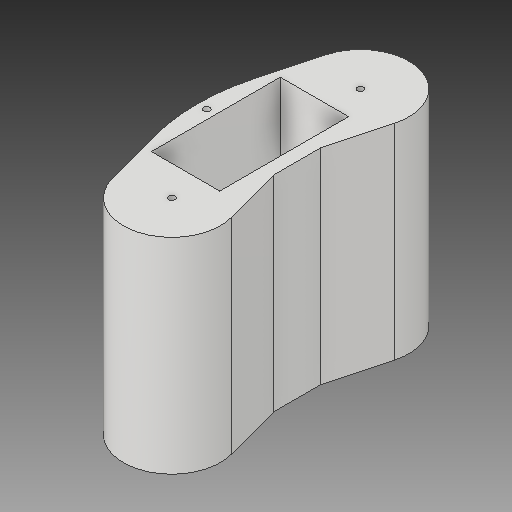
# Autodesk Inventor part: TA001
Saved by Autodesk Inventor 2017 SP1 (Build 210196100, 196)
## iProperties
Created: 2017-09-22
Part Number: TA001
Material: ABS Plastic
Document SubType Name: Modeling
Designer: Zach
Density: 1.06 g/cm^3
Appearance: CR White
Mass: 16966 g
Surface Area: 7360.25 cm^2
Volume: 16005.6 cm^3
Author: Zach
Autodesk Inventor part; units mm, degrees
ref_plane "YZ Plane" through (0, 0, 0) normal (1, 0, 0) x (0, 1, 0)
ref_plane "XZ Plane" through (0, 0, 0) normal (0, 1, 0) x (-1, 0, 0)
ref_plane "XY Plane" through (0, 0, 0) normal (0, 0, 1) x (1, 0, 0)
sketch "Sketch2" plane through (0, 0, 0) normal (0, 1, 0) x (-1, 0, 0)
  circle A0 centre (0, 0) radius 80 construction
  line L0 (77.2741, 20.7055) -> (103.156, -75.8871)
  line L1 (-77.2741, -20.7055) -> (-51.3922, -117.2981)
  line L2 (103.156, -75.8871) -> (-51.3922, -117.2981) construction
  line L3 (103.156, -75.8871) -> (103.156, -235.8871) construction
  line L4 (103.156, -235.8871) -> (-51.3922, -194.476) construction
  line L5 (-51.3922, -117.2981) -> (-51.3922, -194.476)
  circle A1 centre (0, -311.7741) radius 80 construction
  line L6 (-51.3922, -194.476) -> (-77.2741, -291.0686)
  line L7 (103.156, -235.8871) -> (77.2741, -332.4796)
  arc A2 (77.2741, 20.7055) -> (-77.2741, -20.7055) centre (0, 0) ccw
  arc A3 (-77.2741, -291.0686) -> (77.2741, -332.4796) centre (0, -311.7741) ccw
  circle A4 centre (0, 0) radius 5.25
  circle A5 centre (0, -311.7741) radius 5.25
  line L8 (83.156, -49.3871) -> (-29.844, -49.3871)
  line L9 (-29.844, -49.3871) -> (-29.844, -262.3871)
  line L10 (-29.844, -262.3871) -> (83.156, -262.3871)
  line L11 (83.156, -262.3871) -> (83.156, -49.3871)
  arc A6 (103.156, -235.8871) -> (103.156, -75.8871) centre (-201.516, -155.8871) ccw
  circle A7 centre (98.32, -155.8871) radius 5.25
  point P0 (103.156, -155.8871)
  point P1 (83.156, -155.8871)
  dimension "d0" = 160
  dimension "d1" = 100
  dimension "d2" = 100
  dimension "d3" = 160
  dimension "d4" = 160
  dimension "d5" = 160
  dimension "d6" = 75
  dimension "d7" = 75
  dimension "d8" = 160
  dimension "d9" = 100
  dimension "d10" = 100
  dimension "d11" = 10.5
  dimension "d12" = 10.5
  dimension "d13" = 113
  dimension "d14" = 213
  dimension "d15" = 20
  dimension "d39" = 315
  dimension "d40" = 10.5
  dimension "d41" = 15.164
  constraints: 24 end point, 10 point on circle, 8 centre point, 8 tangent, 4 coincident, 2 horizontal alignment, 2 midpoint, 2 parallel, 1 horizontal, 1 perpendicular, 1 vertical
  measures "d0" diameter of A0
  measures "d1" distance of L0.end L0.start
  measures "d2" distance of L1.end L1.start
  measures "d3" distance of L0.end L1.end
  measures "d4" distance of L0.end L3.end
  measures "d5" distance of L3.end L4.end
  measures "d6" angle of L3 L2
  measures "d7" angle of L3 L4
  measures "d8" diameter of A1
  measures "d9" distance of L4.end L6.end
  measures "d10" distance of L3.end L7.end
  measures "d11" diameter of A4
  measures "d12" diameter of A5
  measures "d13" distance of L10.end L9.end
  measures "d14" distance of L9.end L8.end
  measures "d15" distance between parallel lines of L3 L11
  measures "d39" radius of A6
  measures "d40" diameter of A7
  measures "d41" distance from line of L11 A7.centre
extrude "Extrusion1" add sketch "Sketch2" along normal blind 339
sketch "Sketch5" plane through (0, 0, 0) normal (0, -1, 0) x (1, 0, 0)
  circle A0 centre (-98.32, -155.8871) radius 5.25 projected
  circle A1 centre (0, -311.7741) radius 5.25 projected
  circle A2 centre (0, 0) radius 5.25 projected
extrude "Extrusion4" add sketch "Sketch5" against normal blind 5
body "Solid1"
